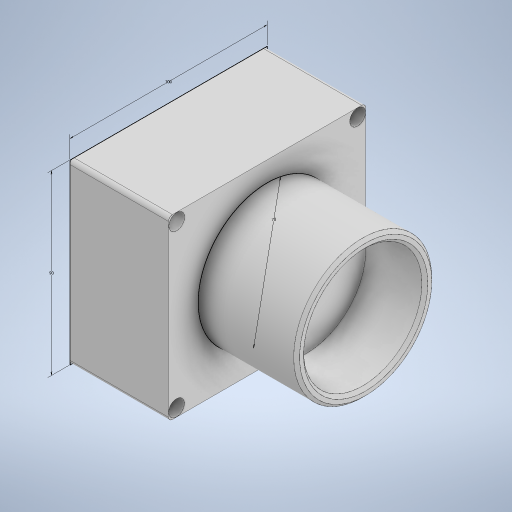
# Autodesk Inventor part: TAREA 1 LAB DINAMICA 1168717
Saved by Autodesk Inventor 2024 (Build 280153000, 153)
## iProperties
Created: 2024-02-06
Part Number: TAREA 1 LAB DINAMICA 1168717
Material: Genérico
Document SubType Name: Modeling
Designer: mariu
Density: 1 g/cm^3
Appearance: Valor por defecto
Author: mariu
Autodesk Inventor part; units mm, degrees
ref_plane "YZ Plane" through (0, 0, 0) normal (1, 0, 0) x (0, 1, 0)
ref_plane "XZ Plane" through (0, 0, 0) normal (0, 1, 0) x (-1, 0, 0)
ref_plane "XY Plane" through (0, 0, 0) normal (0, 0, 1) x (1, 0, 0)
sketch "Boceto1" plane through (0, 0, 0) normal (1, 0, 0) x (0, 1, 0)
  line L0 (-45, -50) -> (45, -50)
  line L1 (45, -50) -> (45, 50)
  line L2 (45, 50) -> (-45, 50)
  line L3 (-45, 50) -> (-45, -50)
  line L4 (-45, -50) -> (45, 50) construction
  line L5 (45, -50) -> (-45, 50) construction
  point P0 (0, 0)
  dimension "d0" = 90
  dimension "d1" = 100
  constraints: 12 end point, 2 midpoint, 2 parallel, 1 horizontal, 1 perpendicular
  measures "d0" distance of L2.end L1.end
  measures "d1" distance of L1.end L0.end
extrude "Extrusión1" add sketch "Boceto1" along normal blind 50
sketch "Boceto2" plane through (50, 0, 0) normal (1, 0, 0) x (0, 0, -1)
  circle A0 centre (0, 0) radius 35
  dimension "d4" = 70
  constraints: 1 centre point, 1 coincident
  measures "d4" diameter of A0
extrude "Extrusión2" add sketch "Boceto2" along normal blind 50
sketch "Boceto3" plane through (100, 0, 0) normal (1, 0, 0) x (0, 0, -1)
  circle A0 centre (0, 0) radius 30
  dimension "d7" = 60
  constraints: 1 centre point, 1 coincident
  measures "d7" diameter of A0
extrude "Extrusión3" cut sketch "Boceto3" against normal blind 30
chamfer "Chaflán1" distance 1.5 angle 45 2 edges at (100, 0, 35) (100, 0, 30)
sketch "Boceto4" plane through (50, 0, 0) normal (1, 0, 0) x (0, 0, -1)
  point P0 (0, 0)
fillet "Empalme1" radius 2 4 edges at (25, 45, 50) (25, -45, 50) (25, 45, -50) (25, -45, -50)
sketch "Boceto5" plane through (50, 0, 0) normal (1, 0, 0) x (0, 0, -1)
  point P0 (0, 0)
  point P1 (-45.8189, 40.8434)
hole "Agujero1" at (50, 40.8434, 45.8189) direction (-1, 0, 0) diameter 8 end through all
sketch "Boceto6" plane through (50, 0, 0) normal (1, 0, 0) x (0, 0, -1)
  line L0 (48, 45) -> (-48, 45) projected
  point P0 (0, 0)
  point P1 (45.9279, 40.9)
  dimension "d21" = 4.1
  measures "d21" distance from line of L0 point (45.928, 40.9)
hole "Agujero2" at (50, 40.9, -45.9279) direction (-1, 0, 0) diameter 8 end through all
sketch "Boceto7" plane through (50, 0, 0) normal (1, 0, 0) x (0, 0, -1)
  line L0 (-48, -45) -> (48, -45) projected
  point P0 (0, 0)
  point P1 (-45.9235, -40.9)
  dimension "d29" = 4.1
  measures "d29" distance from line of L0 point (-45.923, -40.9)
hole "Agujero3" at (50, -40.9, 45.9235) direction (-1, 0, 0) diameter 8 end through all
sketch "Boceto8" plane through (50, 0, 0) normal (1, 0, 0) x (0, 0, -1)
  line L0 (-48, -45) -> (48, -45) projected
  point P0 (0, 0)
  point P1 (45.9358, -40.9)
  dimension "d37" = 4.1
  measures "d37" distance from line of L0 point (45.936, -40.9)
hole "Agujero4" at (50, -40.9, -45.9358) direction (-1, 0, 0) diameter 8 end through all
